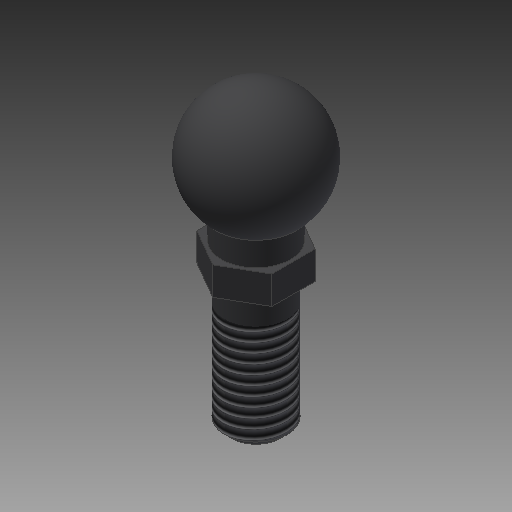
# Autodesk Inventor part: LHSA 10 Body2
Saved by Autodesk Inventor 2018 (Build 220112000, 112)
## iProperties
Category: PARTsolutions
Company: IKO
Created: 2017-10-01
Part Number: LHSA 10 Body2
Catalog Web Link: www.cadenas.de
Description: LHSA B2-
Vendor: IKO
Document SubType Name: Modeling
Designer: psAdmin
Manufacturer: IKO
Mass: 6.06938 g
Surface Area: 21.6199 cm^2
Volume: 6.06938 cm^3
Density: 1 g/cm^3
Material: 一般
Appearance: PSOLRGB-128-128-128
PSOL_IDENT_0: {$CADENAS_DATA\23d-libs\iko\iko_bearings\l_balls\lhsa_body2.prj},169 {VTYP=3D},{NB=LHSA 10 Body2},{L
PSOL_IDENT_1: INA=LHSA 10 Body2},{NN=LHSA B2},{DATE=13.10.2016 10:02:12},{GEOMDATE=05.12.2007 13:50:00},{VERSION=}
PSOL_IDENT_2: ,{LINEID=60},{LINESUBID=-1},{WBVAR=}  {NB=LHSA 10 Body2},{LINA=LHSA 10 Body2},{KT=DUMMY},{IDNR=},{OR
PSOL_IDENT_3: DER=LHSA 10},{RID=G_50},{STDRT=10},{DESCR=LHSA},{TRNUMBER=},{PAST=A},{REST=O},{MASS=106},{S=M10x1.25
PSOL_IDENT_4: },{KDM=8.466},{NDM=10.000},{P1=1.250},{V=10},{D=28},{L=57.0},{L1=43},{L2=23},{SL1=6.5},{W=17},{W1=17
PSOL_IDENT_5: },{W2=17},{D1=15.0},{D2=19},{LL=49.0},{P=12.0},{LL1=16.0},{LL2=21.0},{LL3=17.0},{SDK=19.050},{V1=11.
PSOL_IDENT_6: 0},{D3=12.2475},{D4=21.2001},{D5=26.3},{D6=25.65},{L3=53.8825},{L4=26.1906},{L5=28.5},{L12=30.1645},
PSOL_IDENT_7: {B=8.5},{B1=5.0},{B2=6.5},{B3=11.5},{B4=13.0},{B5=17.5073},{LL4=4.5},{LL5=9.0},{CB=0.0},{CC=0.9},{E=
PSOL_IDENT_8: 0},{F=0.0},{C1=1.1765},{C2=1.0},{R1=5},{R2=34.5114},{R3=15.7},{R4=1.3},{CS=7400},{SS1=8.160},{S1=10}
PSOL_IDENT_9: ,{LX=25},{LX1=28.0},{BL=3},{SC=1}
NN: LHSA B2
NB: LHSA 10 Body2
NBSYN: $ORDER. Body2
LINA: LHSA 10 Body2
ORDER: LHSA 10
RID: G_50
STDRT: 10
DESCR: LHSA
PAST: A
REST: O
MASS: 106
S: M10x1.25
NDM: 10.000
P1: 1.250
V: 10
D: 28
L: 57.0
L1: 43
L2: 23
SL1: 6.5
W: 17
W1: 17
W2: 17
D1: 15.0
D2: 19
LL: 49.0
P: 12.0
LL1: 16.0
LL2: 21.0
LL3: 17.0
SDK: 19.050
V1: 11.0
D3: 12.2475
D4: 21.2001
D5: 26.3
D6: 25.65
L3: 53.8825
L4: 26.1906
L5: 28.5
L12: 30.1645
B: 8.5
B1: 5.0
B2: 6.5
B3: 11.5
B4: 13.0
B5: 17.5073
LL4: 4.5
LL5: 9.0
CB: 0.0
CC: 0.9
E: 0
F: 0.0
C1: 1.1765
C2: 1.0
R1: 5
R2: 34.5114
R3: 15.7
R4: 1.3
CS: 7400
SS1: 8.160
S1: 10
LX: 25
LX1: 28.0
BL: 3
SC: 1
SUPPLIER: IKO
ARTICLENO: LHSA 10 Body2
BOMINFO: LHSA 10 Body2
CREATOR: CADENAS GmbH
Title: LHSA 10 Body2
Author: Cadenas PARTsolutions
Autodesk Inventor part; units mm, degrees
sketch "Sketch_2" plane through (0, 0, 0) normal (0, 0, 1) x (1, 0, 0)
  line L0 (0, -21) -> (0, 25.525)
  arc A0 (6.4595, 9) -> (0, 25.525) centre (0, 16) ccw
  line L1 (6.4595, 9) -> (5.5, 9)
  line L2 (5.5, 9) -> (5.5, 4.5)
  line L3 (5.5, 4.5) -> (7.8, 4.5)
  line L4 (7.8, 4.5) -> (7.8, 0)
  line L5 (7.8, 0) -> (5, 0)
  line L6 (5, 0) -> (5, -20)
  line L7 (5, -20) -> (4, -21)
  line L8 (4, -21) -> (0, -21)
  line L9 (0, -21) -> (0, 25.525)
  constraints: 20 end point, 2 point on circle, 1 centre point
revolve "Revolution1" add sketch "Sketch_2" angle 360 about axis through (0, -21, 0) along (0, -1, 0)
thread "Thread1" size "M10x1.5" class "6g" standard "ISO Metric profile" length 16
sketch "Sketch_3" plane through (0, 4.5, 0) normal (0, 1, 0) x (1, 0, 0)
  line L0 (-12, -12) -> (12, -12)
  line L1 (12, -12) -> (12, 12)
  line L2 (12, 12) -> (-12, 12)
  line L3 (-12, 12) -> (-12, -12)
  line L4 (-6, -3.4641) -> (0, -6.9282)
  line L5 (0, -6.9282) -> (6, -3.4641)
  line L6 (6, -3.4641) -> (6, 3.4641)
  line L7 (6, 3.4641) -> (0, 6.9282)
  line L8 (0, 6.9282) -> (-6, 3.4641)
  line L9 (-6, 3.4641) -> (-6, -3.4641)
  constraints: 20 end point
extrude "Extrusion1" cut sketch "Sketch_3" against normal blind 4.5
ref_plane "IP1_XY" through (0, 16, 0) normal (0, 0, -1) x (1, 0, 0)
ref_plane "IP1_YZ" through (0, 16, 0) normal (1, 0, 0) x (0, -1, 0)
ref_plane "IP1_ZX" through (0, 16, 0) normal (0, -1, 0) x (0, 0, -1)
body "Solid1"
